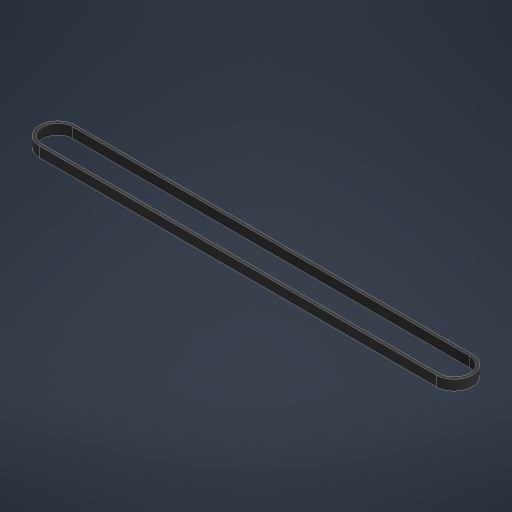
# Autodesk Inventor part: CORL_012_ArmBelt
Saved by Autodesk Inventor 2024.2 (Build 282272000, 272)
## iProperties
Created: 2024-08-05
Part Number: CORL_012_ArmBelt
Material: Rubber, Silicone
Document SubType Name: Modeling
Designer: Bryan
Density: 1.25 g/cm^3
Appearance: Rubber - Black
Author: Bryan
Autodesk Inventor part; units mm, degrees
ref_plane "YZ Plane" through (0, 0, 0) normal (1, 0, 0) x (0, 1, 0)
ref_plane "XZ Plane" through (0, 0, 0) normal (0, 1, 0) x (-1, 0, 0)
ref_plane "XY Plane" through (0, 0, 0) normal (0, 0, 1) x (1, 0, 0)
sketch "Sketch1" plane through (0, 0, 0) normal (0, 1, 0) x (-1, 0, 0)
  circle A0 centre (0, 0) radius 15.9131 construction
  line L0 (0, 0) -> (350.012, 0) construction
  line L1 (350.012, 15.9131) -> (0, 15.9131)
  line L2 (0, -15.9131) -> (350.012, -15.9131)
  arc A1 (350.012, -15.9131) -> (350.012, 15.9131) centre (350.012, 0) ccw
  arc A2 (0, 15.9131) -> (0, -15.9131) centre (0, 0) ccw
  circle A3 centre (350.012, 0) radius 15.9131 construction
  line L3 (0, 13.3731) -> (350.012, 13.3731)
  arc A4 (350.012, -13.3731) -> (350.012, 13.3731) centre (350.012, 0) ccw
  line L4 (350.012, -13.3731) -> (0, -13.3731)
  arc A5 (0, 13.3731) -> (0, -13.3731) centre (0, 0) ccw
  dimension "d0" = 31.8262
  dimension "d1" = 350.012
  dimension "d2" = 31.8262
  dimension "d7" = 2.54
  constraints: 10 end point, 10 point on circle, 6 centre point, 5 tangent, 3 coincident, 1 concentric, 1 horizontal, 3 other
  measures "d0" diameter of A0
  measures "d1" distance of L0.start L0.end
  measures "d2" diameter of A3
  measures "d7" distance between parallel lines of L1 L3
extrude "Extrusion1" add sketch "Sketch1" along normal blind 9
body "Solid1"
